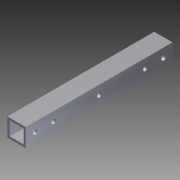
# Autodesk Inventor part: towertopmiddle8inbrace
Saved by Autodesk Inventor 2011 SP1 (Build 150282100, 282)
## iProperties
Created: 2012-01-18
Part Number: towertopmiddle8inbrace
Document SubType Name: Modeling
Designer: Christopher
Density: 1 g/cm^3
Author: Christopher
Autodesk Inventor part; units mm, degrees
ref_plane "YZ Plane" through (0, 0, 0) normal (1, 0, 0) x (0, 1, 0)
ref_plane "XZ Plane" through (0, 0, 0) normal (0, 1, 0) x (-1, 0, 0)
ref_plane "XY Plane" through (0, 0, 0) normal (0, 0, 1) x (1, 0, 0)
sketch "Sketch1" plane through (0, 0, 0) normal (0, 0, 1) x (1, 0, 0)
  line L0 (0, 0) -> (25.4, 0)
  line L1 (25.4, 0) -> (25.4, 25.4)
  line L2 (25.4, 25.4) -> (0, 25.4)
  line L3 (0, 25.4) -> (0, 0)
  line L4 (3.175, 22.225) -> (22.225, 22.225)
  line L5 (22.225, 22.225) -> (22.225, 3.175)
  line L6 (22.225, 3.175) -> (3.175, 3.175)
  line L7 (3.175, 3.175) -> (3.175, 22.225)
  dimension "d0" = 25.4
  dimension "d1" = 25.4
  dimension "d2" = 3.175
  constraints: 16 end point, 4 parallel, 2 perpendicular, 1 horizontal, 3 other
  measures "d0" distance of L1.end L2.end
  measures "d1" distance of L0.end L1.end
  measures "d2" distance between parallel lines of L3 L7
extrude "Extrusion1" add sketch "Sketch1" against normal blind 203.2
sketch "Sketch2" plane through (0, 0, 0) normal (-1, 0, 0) x (0, 0, 1)
  line L0 (-203.2, 25.4) -> (-203.2, 0) projected
  line L1 (0, 25.4) -> (-203.2, 25.4) projected
  line L2 (0, 25.4) -> (0, 0) projected
  point P0 (-190.5, 12.7)
  point P1 (-165.1, 12.7)
  point P2 (-12.7, 12.7)
  point P3 (-38.1, 12.7)
  point P4 (-101.6, 12.7)
  point P5 (-101.6, 12.7)
  dimension "d5" = 12.7
  dimension "d6" = 25.4
  dimension "d7" = 12.7
  dimension "d24" = 12.7
  dimension "d25" = 25.4
  constraints: 1 coincident
  measures "d5" distance from line of L0 point (-190.5, 12.7)
  measures "d6" distance of point (-165.1, 12.7) point (-190.5, 12.7)
  measures "d7" distance from line of L1 point (-190.5, 12.7)
  measures "d24" distance from line of L2 point (-12.7, 12.7)
  measures "d25" distance of point (-12.7, 12.7) point (-38.1, 12.7)
hole "Hole1" at (0, 12.7, -190.5) at (0, 12.7, -165.1) at (0, 12.7, -38.1) at (0, 12.7, -12.7) at (0, 12.7, -101.6) direction (1, 0, 0) diameter 6.35 depth 25.4 tip angle 118
body "Solid1"
